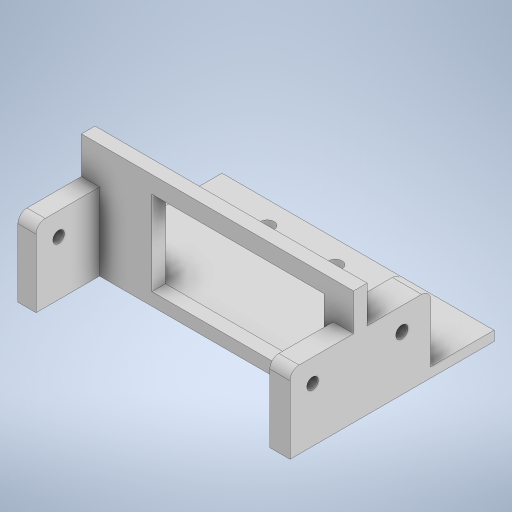
# Autodesk Inventor part: Base-Configurable-Dribler
Saved by Autodesk Inventor 2024.2 (Build 282272000, 272)
## iProperties
Created: 2023-12-01
Part Number: Base-Configurable-Dribler
Material: Generic
Document SubType Name: Modeling
Designer: felip
Density: 1 g/cm^3
Appearance: Default
Author: felip
Autodesk Inventor part; units mm, degrees
ref_plane "YZ Plane" through (0, 0, 0) normal (1, 0, 0) x (0, 1, 0)
ref_plane "XZ Plane" through (0, 0, 0) normal (0, 1, 0) x (-1, 0, 0)
ref_plane "XY Plane" through (0, 0, 0) normal (0, 0, 1) x (1, 0, 0)
sketch "Sketch1" plane through (0, 0, 0) normal (0, 1, 0) x (-1, 0, 0)
  line L0 (0, 0) -> (-30, 0)
  line L1 (-30, 0) -> (30, 0)
  line L2 (30, 0) -> (30, -15)
  line L3 (30, -15) -> (-30, -15)
  line L4 (-30, -15) -> (-30, 15)
  line L5 (-30, 15) -> (30, 15)
  line L6 (30, 15) -> (30, -15)
  line L7 (0, 0) -> (0, -10)
  line L8 (0, -10) -> (-15, -10)
  line L9 (0, -10) -> (15, -10)
  circle A0 centre (15, -10) radius 1.5
  circle A1 centre (0, -10) radius 1.5
  circle A2 centre (-15, -10) radius 1.5
  dimension "d0" = 30
  dimension "d1" = 60
  dimension "d2" = 15
  dimension "d3" = 30
  dimension "d4" = 10
  dimension "d5" = 15
  dimension "d6" = 15
  dimension "d7" = 3
  dimension "d8" = 3
  dimension "d9" = 3
  constraints: 20 end point, 3 centre point, 3 coincident, 3 horizontal, 2 parallel, 2 perpendicular, 2 vertical, 1 point on line
  measures "d0" distance of L0.start L0.end
  measures "d1" distance of L0.end L1.end
  measures "d2" distance of L1.end L2.end
  measures "d3" distance of L3.end L4.end
  measures "d4" distance of L0.start L7.end
  measures "d5" distance of L7.end L8.end
  measures "d6" distance of L7.end L9.end
  measures "d7" diameter of A0
  measures "d8" diameter of A1
  measures "d9" diameter of A2
extrude "Extrusion1" add sketch "Sketch1" along normal blind 2
sketch "Sketch2" plane through (0, 2, 0) normal (0, 1, 0) x (1, 0, 0)
  line L0 (-30, -15) -> (30, -15) projected
  line L1 (-30, 15) -> (-30, -15) projected
  line L2 (30, -15) -> (-30, -15)
  line L3 (-30, -15) -> (-30, -13)
  line L4 (-30, -13) -> (30, -13)
  line L5 (30, -13) -> (30, -15)
  point P0 (0, 0)
  dimension "d12" = 2
  constraints: 8 end point, 2 parallel, 1 horizontal, 1 perpendicular, 1 point on line
  measures "d12" distance of L2.end L3.end
extrude "Extrusion2" add sketch "Sketch2" along normal blind 28
sketch "Sketch3" plane through (30, 2, 13) normal (0, 0, -1) x (-1, 0, 0)
  line L0 (28.5, 0) -> (31.5, 0) projected
  line L1 (0, 0) -> (0, 28) projected
  line L2 (4.4524, 13.5) -> (4.4524, 14.95)
  line L3 (0, 14) -> (2, 14)
  line L4 (4.4524, 14.95) -> (4.4524, 5.8)
  line L5 (4.4524, 14.95) -> (4.4524, 24.2)
  line L6 (4.4524, 5.8) -> (44.4524, 5.8)
  line L7 (44.4524, 5.8) -> (44.4524, 24.2)
  line L8 (44.4524, 24.2) -> (4.4524, 24.2)
  line L9 (4.4524, 24.2) -> (4.4524, 5.8)
  line L10 (0, 0) -> (60, 0) projected
  point P0 (30, -2)
  point P1 (4.4524, 24.2)
  point P2 (4.4524, 15)
  dimension "d42" = 2
  dimension "d43" = 9.15
  dimension "d44" = 9.25
  dimension "d45" = 40
  dimension "d53" = 15
  dimension "d71" = 18.4
  constraints: 16 end point, 2 midpoint, 2 parallel, 2 vertical, 1 horizontal, 1 perpendicular
  measures "d42" distance of L3.start L3.end
  measures "d43" distance of L2.end L4.end
  measures "d44" distance of L2.end L5.end
  measures "d45" distance of L8.end L7.end
  measures "d53" distance from line of point (4.452, 15) L10
  measures "d71" distance between parallel lines of L8 L6
sketch "Sketch4" plane through (30, 2, 13) normal (0, 0, -1) x (-1, 0, 0)
  line L0 (28.5, 0) -> (31.5, 0) projected
  line L1 (30, 0) -> (30, 15)
  line L2 (42, 9.5) -> (4.4524, 9.5) projected
  line L3 (30, 0) -> (45, 0) construction
  line L4 (30, 15) -> (0, 15)
  line L5 (0, 15) -> (0, 10)
  line L6 (0, 10) -> (4, 10)
  line L7 (4, 10) -> (4, 20)
  line L8 (4, 20) -> (0, 20)
  line L9 (0, 20) -> (0, 10)
  point P0 (30, -2)
  point P1 (4, 15)
  dimension "d20" = 15
  dimension "d21" = 90
  dimension "d22" = 5
  dimension "d24" = 4
  dimension "d51" = 5
  constraints: 16 end point, 3 perpendicular, 2 horizontal, 2 parallel, 1 midpoint
  measures "d20" distance of L1.start L1.end
  measures "d21" angle of L3 L1
  measures "d22" distance of L4.end L5.end
  measures "d24" distance of L8.end L7.end
  measures "d51" distance between parallel lines of L8 L4
extrude "Extrusion4" add sketch "Sketch4" along normal blind 14
sketch "Sketch5" plane through (30, 0, 15) normal (1, 0, 0) x (0, 0, -1)
  line L0 (2, 22) -> (2, 30) projected
  line L1 (2, 22) -> (2, 17)
  line L2 (2, 22) -> (2, 12) projected
  line L3 (2, 17) -> (9.668, 17)
  circle A0 centre (9.668, 17) radius 1.35
  point P0 (15, 0)
  dimension "d27" = 5
  dimension "d28" = 7.668
  dimension "d29" = 2.7
  constraints: 4 end point, 1 centre point, 1 coincident, 1 midpoint, 1 perpendicular
  measures "d27" distance of L0.start L1.end
  measures "d28" distance of L1.end L3.end
  measures "d29" diameter of A0
extrude "Extrusion5" cut sketch "Sketch5" against normal blind 10
sketch "Sketch6" plane through (30, 0, 15) normal (1, 0, 0) x (0, 0, -1)
  circle A0 centre (9.668, 17) radius 1.35 projected
  line L0 (9.668, 17) -> (-10.032, 17)
  line L1 (2, 22) -> (16, 22) projected
  line L2 (2, 22) -> (0, 22)
  line L3 (0, 0) -> (0, 30) projected
  line L4 (2, 12) -> (16, 12) projected
  line L5 (2, 12) -> (0, 12)
  line L6 (0, 22) -> (-15, 22)
  line L7 (-15, 22) -> (-15, 5)
  line L8 (-15, 5) -> (0, 5)
  line L9 (0, 5) -> (0, 22)
  circle A1 centre (-10.032, 17) radius 1.27
  point P0 (15, 0)
  point P1 (0, 5)
  dimension "d32" = 19.7
  dimension "d33" = 15
  dimension "d48" = 2.54
  dimension "d49" = 5
  dimension "d74" = 5
  constraints: 14 end point, 4 horizontal, 2 parallel, 1 centre point, 1 coincident, 1 perpendicular, 1 point on line
  measures "d32" distance of L0.start L0.end
  measures "d33" distance of L8.end L7.end
  measures "d48" diameter of A1
  measures "d49" distance between parallel lines of L6 L0
  measures "d74" distance from line of L3.start L8
extrude "Extrusion6" add sketch "Sketch6" against normal blind 60 contours L8 L7 L6 L3
sketch "Sketch7" plane through (30, 5, 30) normal (0, 0, 1) x (1, 0, 0)
  line L0 (-60, 17) -> (-60, 25) projected
  line L1 (0, 0) -> (-60, 0) projected
  line L2 (-60, 17) -> (0, 17)
  line L3 (0, 17) -> (0, 0)
  line L4 (0, 0) -> (-60, 0)
  line L5 (-60, 0) -> (-60, 17)
  line L6 (-60, 8.5) -> (-56, 8.5)
  line L7 (0, 8.5) -> (-4, 8.5)
  line L8 (-56, 8.5) -> (-56, 17)
  line L9 (-56, 17) -> (-4, 17)
  line L10 (-4, 17) -> (-4, 0)
  line L11 (-4, 0) -> (-56, 0)
  line L12 (-56, 0) -> (-56, 17)
  point P0 (-30, -5)
  point P1 (-56, 8.5)
  point P2 (-56, 0)
  point P3 (-4, 0)
  point P4 (-4, 17)
  dimension "d36" = 4
  dimension "d37" = 4
  dimension "d50" = 4
  constraints: 22 end point, 4 horizontal, 4 parallel, 3 perpendicular, 2 midpoint, 2 point on line
  measures "d36" distance of L6.start L6.end
  measures "d37" distance of L7.start L7.end
  measures "d50" distance between parallel lines of L10 L3
extrude "Extrusion7" cut sketch "Sketch7" against normal blind 15 contours L1 L12 L8 L2 L10
fillet "Fillet1" radius 2 2 edges at (28, 22, -1) (28, 12, -1)
extrude "Extrusion8" cut sketch "Sketch3" against normal blind 12
thicken "Thicken1" operation add thickness 5.85 both sides no extend neighbours no toward (0, 1, 0) faces at (-0.0603, 2, 5.8297)
sketch "Sketch8" plane through (30, 0, 15) normal (1, 0, 0) x (0, 0, -1)
  line L0 (2, 7.8) -> (0, 7.8) projected
  arc A0 (14, 12) -> (16, 14) centre (14, 14) ccw projected
  line L1 (2, 7.85) -> (16, 7.85)
  line L2 (16, 7.85) -> (16, 14)
  line L3 (16, 14) -> (2, 14)
  line L4 (2, 14) -> (2, 7.85)
  point P0 (15, 0)
  point P1 (0, 7.85)
  constraints: 8 end point, 2 parallel, 1 horizontal, 1 perpendicular, 1 other
extrude "Extrusion9" add sketch "Sketch8" against normal blind 4
thicken "Thicken2" operation add thickness 1 both sides no extend neighbours no toward (0, 0, 1) faces at (-4.8175, 2.6, 15)
thicken "Thicken3" operation add thickness 0.15 both sides no extend neighbours no toward (0, 1, 0) faces at (-10, 30, 14)
thicken "Thicken4" operation add thickness 0.452 both sides no extend neighbours no toward (-1, 0, 0) faces at (26, 10.4533, 5.8316)
thicken "Thicken5" operation add thickness 0.452 both sides no extend neighbours no toward (-1, 0, 0) faces at (26, 8.5798, 23.6263)
thicken "Thicken6" operation add thickness 2 both sides no extend neighbours no toward (-1, 0, 0) faces at (25.5476, 13.95, 15)
thicken "Thicken7" operation add thickness 2 both sides no extend neighbours no toward (-1, 0, 0) faces at (25.548, 10.4533, 5.8316)
sketch "Sketch9" plane through (0, 0, 0) normal (0, -1, 0) x (1, 0, 0)
  line L0 (-30, -15) -> (-30, 16) projected
  line L1 (-30, 16) -> (30, 16) projected
  line L2 (-30, -15) -> (30, -15)
  line L3 (30, -15) -> (30, 16)
  line L4 (30, 16) -> (-30, 16)
  line L5 (-30, 16) -> (-30, -15)
  point P0 (0, 0)
  constraints: 8 end point, 2 parallel, 1 horizontal, 1 perpendicular
extrude "Extrusion10" cut sketch "Sketch9" against normal blind 5
fillet "Fillet3" radius 2 2 edges at (27.774, 22, 30) (-28, 22, 30)
sketch "Sketch10" plane through (-30, 7.85, -15) normal (0, 1, 0) x (1, 0, 0)
  line L0 (15.5476, -28) -> (0, -28) projected
  line L1 (0, 0) -> (0, -28) projected
  line L2 (0, -28) -> (0, 0)
  line L3 (60, -14) -> (60, 0) projected
  line L4 (0, 0) -> (60, 0)
  line L5 (60, 0) -> (60, -14)
  line L6 (53.548, -28) -> (53.548, -14) projected
  line L7 (60, -14) -> (53.548, -14)
  line L8 (53.548, -14) -> (53.548, -28)
  line L9 (53.548, -28) -> (0, -28)
  point P0 (30, -15)
  constraints: 12 end point, 4 perpendicular, 1 collinear, 1 vertical
extrude "Extrusion11" cut sketch "Sketch10" against normal blind 0.7
sketch "Sketch11" plane through (-14.4524, 26.2, 13) normal (0, -1, 0) x (1, 0, 0)
  line L0 (38, 0) -> (0, 0) projected
  line L1 (0, 0) -> (38, 0)
  line L2 (38, 0) -> (38, 3)
  line L3 (38, 3) -> (0, 3)
  line L4 (0, 3) -> (0, 0)
  point P0 (14.4524, -13)
  constraints: 8 end point, 2 parallel, 1 horizontal, 1 perpendicular
extrude "Extrusion12" cut sketch "Sketch11" against normal blind 0.2
body "Solid1"
